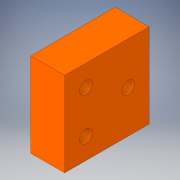
# Autodesk Inventor part: tOPgRIPPERcLAMP
Saved by Autodesk Inventor 2019 (Build 230136000, 136)
## iProperties
Created: 2019-10-03
Part Number: tOPgRIPPERcLAMP
Material: Generic
Document SubType Name: Modeling
Designer: james
Density: 1 g/cm^3
Appearance: Default(1)
Author: james
Autodesk Inventor part; units mm, degrees
ref_plane "YZ Plane" through (0, 0, 0) normal (1, 0, 0) x (0, 1, 0)
ref_plane "XZ Plane" through (0, 0, 0) normal (0, 1, 0) x (-1, 0, 0)
ref_plane "XY Plane" through (0, 0, 0) normal (0, 0, 1) x (1, 0, 0)
sketch "Sketch1" plane through (0, 0, 0) normal (1, 0, 0) x (0, 1, 0)
  line L0 (15.8212, 35.7681) -> (-9.5788, 35.7681)
  line L1 (-9.5788, 35.7681) -> (-9.5788, 10.3681)
  line L2 (-9.5788, 10.3681) -> (15.8212, 10.3681)
  line L3 (15.8212, 10.3681) -> (15.8212, 35.7681)
  point P0 (0, 0)
  dimension "d0" = 25.4
  dimension "d1" = 25.4
  constraints: 8 end point, 2 parallel, 1 horizontal, 1 perpendicular
  measures "d0" distance of L2.end L0.start
  measures "d1" distance of L1.end L2.end
extrude "Extrusion1" add sketch "Sketch1" along normal blind 10.16
sketch "Sketch2" plane through (10.16, 0, 0) normal (1, 0, 0) x (0, 0, -1)
  line L0 (-35.7681, 15.8212) -> (-35.7681, -9.5788) projected
  line L1 (-10.3681, 15.8212) -> (-35.7681, 15.8212) projected
  line L2 (-35.7681, -9.5788) -> (-10.3681, -9.5788) projected
  point P0 (0, 0)
  point P1 (-29.4181, 9.4712)
  point P2 (-29.4181, -3.2288)
  point P3 (-16.7181, 3.1212)
  dimension "d4" = 19.05
  dimension "d5" = 12.7
  dimension "d6" = 6.35
  dimension "d7" = 6.35
  dimension "d8" = 0
  dimension "d9" = 6.35
  measures "d4" distance from line of L0 point (-16.718, 3.121)
  measures "d5" distance from line of L1 point (-16.718, 3.121)
  measures "d6" distance from line of L1 point (-29.418, 9.471)
  measures "d7" distance from line of L0 point (-29.418, 9.471)
  measures "d8" horizontal distance of point (-29.418, 9.471) point (-29.418, -3.229)
  measures "d9" distance from line of L2 point (-29.418, -3.229)
hole "Hole1" at (10.16, 9.4712, 29.4181) at (10.16, -3.2288, 29.4181) at (10.16, 3.1212, 16.7181) direction (-1, 0, 0) diameter 3.81 depth 10.9728 tip angle 118.188 clearance for "Flat Head Machine Screw (82)" size "#6" standard "Ansi Unified Screw Threads"
body "Solid1"
